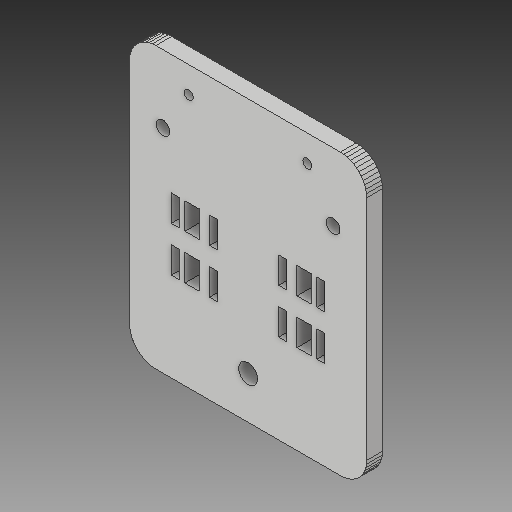
# Autodesk Inventor part: X-Axis-End-Plate
Saved by Autodesk Inventor 2018 (Build 220112000, 112)
## iProperties
Created: 2016-07-20
Part Number: X-Axis-End-Plate
Material: Generic
Document SubType Name: Modeling
Designer: User
Density: 1 g/cm^3
Appearance: Default
Mass: 53.5159 g
Surface Area: 225.376 cm^2
Volume: 53.5159 cm^3
Author: User
Autodesk Inventor part; units mm, degrees
ref_plane "YZ Plane" through (0, 0, 0) normal (1, 0, 0) x (0, 1, 0)
ref_plane "XZ Plane" through (0, 0, 0) normal (0, 1, 0) x (-1, 0, 0)
ref_plane "XY Plane" through (0, 0, 0) normal (0, 0, 1) x (1, 0, 0)
sketch "Sketch1" plane through (0, 0, 0) normal (0, 0, 1) x (1, 0, 0)
  line L0 (481.879114, 151.794374) -> (481.879114, 141.794403)
  line L1 (481.879114, 141.794403) -> (484.879103, 141.794403)
  line L2 (484.879103, 141.794403) -> (484.879103, 151.794374)
  line L3 (484.879103, 151.794374) -> (481.879114, 151.794374)
  line L4 (481.879114, 134.794399) -> (481.879114, 124.794385)
  line L5 (481.879114, 124.794385) -> (484.879103, 124.794385)
  line L6 (484.879103, 124.794385) -> (484.879103, 134.794399)
  line L7 (484.879103, 134.794399) -> (481.879114, 134.794399)
  line L8 (467.379094, 134.794399) -> (467.379094, 124.794385)
  line L9 (467.379094, 124.794385) -> (470.379127, 124.794385)
  line L10 (470.379127, 124.794385) -> (470.379127, 134.794399)
  line L11 (470.379127, 134.794399) -> (467.379094, 134.794399)
  line L12 (472.529125, 134.794399) -> (472.529125, 124.794385)
  line L13 (472.529125, 124.794385) -> (477.929139, 124.794385)
  line L14 (477.929139, 124.794385) -> (477.929139, 134.794399)
  line L15 (477.929139, 134.794399) -> (472.529125, 134.794399)
  line L16 (472.529125, 151.794374) -> (472.529125, 141.794403)
  line L17 (472.529125, 141.794403) -> (477.929139, 141.794403)
  line L18 (477.929139, 141.794403) -> (477.929139, 151.794374)
  line L19 (477.929139, 151.794374) -> (472.529125, 151.794374)
  line L20 (467.379094, 151.794374) -> (467.379094, 141.794403)
  line L21 (467.379094, 141.794403) -> (470.379127, 141.794403)
  line L22 (470.379127, 141.794403) -> (470.379127, 151.794374)
  line L23 (470.379127, 151.794374) -> (467.379094, 151.794374)
  line L24 (541.393546, 188.55966) -> (541.13835, 189.842592)
  line L25 (541.13835, 189.842592) -> (540.717954, 191.081259)
  line L26 (540.717954, 191.081259) -> (540.139367, 192.254387)
  line L27 (540.139367, 192.254387) -> (539.412654, 193.342024)
  line L28 (539.412654, 193.342024) -> (538.550163, 194.325482)
  line L29 (538.550163, 194.325482) -> (537.566754, 195.187911)
  line L30 (537.566754, 195.187911) -> (536.479128, 195.914617)
  line L31 (536.479128, 195.914617) -> (535.30593, 196.493238)
  line L32 (535.30593, 196.493238) -> (534.067263, 196.913635)
  line L33 (534.067263, 196.913635) -> (532.784356, 197.168825)
  line L34 (532.784356, 197.168825) -> (531.479096, 197.254393)
  line L35 (531.479096, 197.254393) -> (461.479063, 197.254393)
  line L36 (461.479063, 197.254393) -> (460.173846, 197.168827)
  line L37 (460.173846, 197.168827) -> (458.890898, 196.913628)
  line L38 (458.890898, 196.913628) -> (457.652231, 196.493231)
  line L39 (457.652231, 196.493231) -> (456.479102, 195.914644)
  line L40 (456.479102, 195.914644) -> (455.391476, 195.187938)
  line L41 (455.391476, 195.187938) -> (454.408051, 194.325477)
  line L42 (454.408051, 194.325477) -> (453.545572, 193.34201)
  line L43 (453.545572, 193.34201) -> (452.818872, 192.254393)
  line L44 (452.818872, 192.254393) -> (452.240268, 191.081231)
  line L45 (452.240268, 191.081231) -> (451.81988, 189.84259)
  line L46 (451.81988, 189.84259) -> (451.564685, 188.559658)
  line L47 (451.564685, 188.559658) -> (451.479117, 187.254397)
  line L48 (451.479117, 187.254397) -> (451.479117, 100.994374)
  line L49 (451.479117, 100.994374) -> (451.564685, 99.689135)
  line L50 (451.564685, 99.689135) -> (451.81988, 98.406203)
  line L51 (451.81988, 98.406203) -> (452.240268, 97.167562)
  line L52 (452.240268, 97.167562) -> (452.818872, 95.994399)
  line L53 (452.818872, 95.994399) -> (453.545572, 94.906782)
  line L54 (453.545572, 94.906782) -> (454.408051, 93.923337)
  line L55 (454.408051, 93.923337) -> (455.391496, 93.060877)
  line L56 (455.391496, 93.060877) -> (456.479122, 92.334171)
  line L57 (456.479122, 92.334171) -> (457.652251, 91.755584)
  line L58 (457.652251, 91.755584) -> (458.890911, 91.335189)
  line L59 (458.890911, 91.335189) -> (460.173864, 91.07999)
  line L60 (460.173864, 91.07999) -> (461.47908, 90.994425)
  line L61 (461.47908, 90.994425) -> (531.479114, 90.994425)
  line L62 (531.479114, 90.994425) -> (532.784373, 91.079994)
  line L63 (532.784373, 91.079994) -> (534.067285, 91.335185)
  line L64 (534.067285, 91.335185) -> (535.306039, 91.755612)
  line L65 (535.306039, 91.755612) -> (536.479237, 92.334233)
  line L66 (536.479237, 92.334233) -> (537.566863, 93.060939)
  line L67 (537.566863, 93.060939) -> (538.550274, 93.923388)
  line L68 (538.550274, 93.923388) -> (539.412743, 94.906843)
  line L69 (539.412743, 94.906843) -> (540.139456, 95.99448)
  line L70 (540.139456, 95.99448) -> (540.71798, 97.167481)
  line L71 (540.71798, 97.167481) -> (541.13843, 98.406304)
  line L72 (541.13843, 98.406304) -> (541.393625, 99.689236)
  line L73 (541.393625, 99.689236) -> (541.47915, 100.993841)
  line L74 (541.47915, 100.993841) -> (541.47915, 187.253864)
  line L75 (541.47915, 187.253864) -> (541.393546, 188.55966)
  line L76 (466.594249, 172.241537) -> (466.344494, 172.844478)
  line L77 (466.344494, 172.844478) -> (465.947221, 173.362246)
  line L78 (465.947221, 173.362246) -> (465.429438, 173.759515)
  line L79 (465.429438, 173.759515) -> (464.826482, 174.009293)
  line L80 (464.826482, 174.009293) -> (464.17945, 174.094495)
  line L81 (464.17945, 174.094495) -> (463.532378, 174.00927)
  line L82 (463.532378, 174.00927) -> (462.929452, 173.759522)
  line L83 (462.929452, 173.759522) -> (462.411649, 173.362223)
  line L84 (462.411649, 173.362223) -> (462.014386, 172.844447)
  line L85 (462.014386, 172.844447) -> (461.764617, 172.241512)
  line L86 (461.764617, 172.241512) -> (461.679408, 171.594428)
  line L87 (461.679408, 171.594428) -> (461.764626, 170.947406)
  line L88 (461.764626, 170.947406) -> (462.014395, 170.344429)
  line L89 (462.014395, 170.344429) -> (462.411658, 169.826674)
  line L90 (462.411658, 169.826674) -> (462.929469, 169.429385)
  line L91 (462.929469, 169.429385) -> (463.532388, 169.179622)
  line L92 (463.532388, 169.179622) -> (464.179462, 169.094414)
  line L93 (464.179462, 169.094414) -> (464.826492, 169.179633)
  line L94 (464.826492, 169.179633) -> (465.429455, 169.429396)
  line L95 (465.429455, 169.429396) -> (465.94723, 169.826675)
  line L96 (465.94723, 169.826675) -> (466.344482, 170.344437)
  line L97 (466.344482, 170.344437) -> (466.594267, 170.947409)
  line L98 (466.594267, 170.947409) -> (466.679473, 171.594468)
  line L99 (466.679473, 171.594468) -> (466.594249, 172.241537)
  line L100 (475.620434, 187.694279) -> (475.450597, 188.104291)
  line L101 (475.450597, 188.104291) -> (475.180424, 188.456408)
  line L102 (475.180424, 188.456408) -> (474.828325, 188.726555)
  line L103 (474.828325, 188.726555) -> (474.418362, 188.896385)
  line L104 (474.418362, 188.896385) -> (473.97834, 188.954328)
  line L105 (473.97834, 188.954328) -> (473.538405, 188.896385)
  line L106 (473.538405, 188.896385) -> (473.128364, 188.726535)
  line L107 (473.128364, 188.726535) -> (472.77627, 188.456381)
  line L108 (472.77627, 188.456381) -> (472.506125, 188.104284)
  line L109 (472.506125, 188.104284) -> (472.336277, 187.694277)
  line L110 (472.336277, 187.694277) -> (472.27834, 187.254297)
  line L111 (472.27834, 187.254297) -> (472.336289, 186.814319)
  line L112 (472.336289, 186.814319) -> (472.506134, 186.404289)
  line L113 (472.506134, 186.404289) -> (472.77627, 186.05222)
  line L114 (472.77627, 186.05222) -> (473.128369, 185.782073)
  line L115 (473.128369, 185.782073) -> (473.538405, 185.612213)
  line L116 (473.538405, 185.612213) -> (473.978345, 185.554281)
  line L117 (473.978345, 185.554281) -> (474.418368, 185.612235)
  line L118 (474.418368, 185.612235) -> (474.828336, 185.782055)
  line L119 (474.828336, 185.782055) -> (475.180429, 186.052209)
  line L120 (475.180429, 186.052209) -> (475.450574, 186.404304)
  line L121 (475.450574, 186.404304) -> (475.620429, 186.81433)
  line L122 (475.620429, 186.81433) -> (475.678374, 187.254369)
  line L123 (475.678374, 187.254369) -> (475.620434, 187.694279)
  line L124 (499.931821, 107.918802) -> (499.575329, 108.779425)
  line L125 (499.575329, 108.779425) -> (499.008238, 109.518518)
  line L126 (499.008238, 109.518518) -> (498.269158, 110.085575)
  line L127 (498.269158, 110.085575) -> (497.408529, 110.442096)
  line L128 (497.408529, 110.442096) -> (496.484906, 110.56372)
  line L129 (496.484906, 110.56372) -> (495.561371, 110.442083)
  line L130 (495.561371, 110.442083) -> (494.700696, 110.085568)
  line L131 (494.700696, 110.085568) -> (493.9616, 109.518475)
  line L132 (493.9616, 109.518475) -> (493.394525, 108.779372)
  line L133 (493.394525, 108.779372) -> (493.03801, 107.918758)
  line L134 (493.03801, 107.918758) -> (492.916389, 106.995156)
  line L135 (492.916389, 106.995156) -> (493.038034, 106.071557)
  line L136 (493.038034, 106.071557) -> (493.394527, 105.210934)
  line L137 (493.394527, 105.210934) -> (493.961618, 104.471842)
  line L138 (493.961618, 104.471842) -> (494.700725, 103.904764)
  line L139 (494.700725, 103.904764) -> (495.561391, 103.548228)
  line L140 (495.561391, 103.548228) -> (496.484929, 103.426615)
  line L141 (496.484929, 103.426615) -> (497.408549, 103.548263)
  line L142 (497.408549, 103.548263) -> (498.269187, 103.904762)
  line L143 (498.269187, 103.904762) -> (499.008255, 104.471834)
  line L144 (499.008255, 104.471834) -> (499.575331, 105.210938)
  line L145 (499.575331, 105.210938) -> (499.931846, 106.071552)
  line L146 (499.931846, 106.071552) -> (500.05347, 106.995179)
  line L147 (500.05347, 106.995179) -> (499.931821, 107.918802)
  line L148 (508.079065, 151.794374) -> (508.079065, 141.794403)
  line L149 (508.079065, 141.794403) -> (511.07914, 141.794403)
  line L150 (511.07914, 141.794403) -> (511.07914, 151.794374)
  line L151 (511.07914, 151.794374) -> (508.079065, 151.794374)
  line L152 (520.621398, 187.694369) -> (520.45156, 188.104381)
  line L153 (520.45156, 188.104381) -> (520.181388, 188.456498)
  line L154 (520.181388, 188.456498) -> (519.829289, 188.726645)
  line L155 (519.829289, 188.726645) -> (519.419326, 188.896475)
  line L156 (519.419326, 188.896475) -> (518.979304, 188.954417)
  line L157 (518.979304, 188.954417) -> (518.539284, 188.896463)
  line L158 (518.539284, 188.896463) -> (518.129316, 188.726644)
  line L159 (518.129316, 188.726644) -> (517.777223, 188.45649)
  line L160 (517.777223, 188.45649) -> (517.507083, 188.1044)
  line L161 (517.507083, 188.1044) -> (517.337241, 187.694408)
  line L162 (517.337241, 187.694408) -> (517.279303, 187.254423)
  line L163 (517.279303, 187.254423) -> (517.337253, 186.814439)
  line L164 (517.337253, 186.814439) -> (517.507092, 186.404425)
  line L165 (517.507092, 186.404425) -> (517.777228, 186.052355)
  line L166 (517.777228, 186.052355) -> (518.129326, 185.782208)
  line L167 (518.129326, 185.782208) -> (518.539289, 185.612378)
  line L168 (518.539289, 185.612378) -> (518.979314, 185.554435)
  line L169 (518.979314, 185.554435) -> (519.419337, 185.61239)
  line L170 (519.419337, 185.61239) -> (519.829305, 185.782209)
  line L171 (519.829305, 185.782209) -> (520.181398, 186.052363)
  line L172 (520.181398, 186.052363) -> (520.451543, 186.404459)
  line L173 (520.451543, 186.404459) -> (520.621398, 186.814485)
  line L174 (520.621398, 186.814485) -> (520.679336, 187.25447)
  line L175 (520.679336, 187.25447) -> (520.621398, 187.694369)
  line L176 (522.579127, 134.794399) -> (522.579127, 124.794385)
  line L177 (522.579127, 124.794385) -> (525.579116, 124.794385)
  line L178 (525.579116, 124.794385) -> (525.579116, 134.794399)
  line L179 (525.579116, 134.794399) -> (522.579127, 134.794399)
  line L180 (522.579127, 151.794374) -> (522.579127, 141.794403)
  line L181 (522.579127, 141.794403) -> (525.579116, 141.794403)
  line L182 (525.579116, 141.794403) -> (525.579116, 151.794374)
  line L183 (525.579116, 151.794374) -> (522.579127, 151.794374)
  line L184 (515.029114, 134.794399) -> (515.029114, 124.794385)
  line L185 (515.029114, 124.794385) -> (520.429129, 124.794385)
  line L186 (520.429129, 124.794385) -> (520.429129, 134.794399)
  line L187 (520.429129, 134.794399) -> (515.029114, 134.794399)
  line L188 (531.194569, 172.24152) -> (530.944815, 172.844461)
  line L189 (530.944815, 172.844461) -> (530.547526, 173.36225)
  line L190 (530.547526, 173.36225) -> (530.029743, 173.759518)
  line L191 (530.029743, 173.759518) -> (529.426786, 174.009297)
  line L192 (529.426786, 174.009297) -> (528.779755, 174.094499)
  line L193 (528.779755, 174.094499) -> (528.132682, 174.009274)
  line L194 (528.132682, 174.009274) -> (527.529793, 173.759541)
  line L195 (527.529793, 173.759541) -> (527.011991, 173.362242)
  line L196 (527.011991, 173.362242) -> (526.614712, 172.844445)
  line L197 (526.614712, 172.844445) -> (526.364949, 172.241525)
  line L198 (526.364949, 172.241525) -> (526.279744, 171.594475)
  line L199 (526.279744, 171.594475) -> (526.364963, 170.947448)
  line L200 (526.364963, 170.947448) -> (526.614726, 170.344486)
  line L201 (526.614726, 170.344486) -> (527.012005, 169.82671)
  line L202 (527.012005, 169.82671) -> (527.529815, 169.429421)
  line L203 (527.529815, 169.429421) -> (528.132698, 169.179673)
  line L204 (528.132698, 169.179673) -> (528.779773, 169.094466)
  line L205 (528.779773, 169.094466) -> (529.426802, 169.179685)
  line L206 (529.426802, 169.179685) -> (530.029765, 169.429448)
  line L207 (530.029765, 169.429448) -> (530.54754, 169.826726)
  line L208 (530.54754, 169.826726) -> (530.944744, 170.344426)
  line L209 (530.944744, 170.344426) -> (531.194529, 170.947397)
  line L210 (531.194529, 170.947397) -> (531.279764, 171.594678)
  line L211 (531.279764, 171.594678) -> (531.194569, 172.24152)
  line L212 (508.079065, 134.794399) -> (508.079065, 124.794385)
  line L213 (508.079065, 124.794385) -> (511.07914, 124.794385)
  line L214 (511.07914, 124.794385) -> (511.07914, 134.794399)
  line L215 (511.07914, 134.794399) -> (508.079065, 134.794399)
  line L216 (515.029114, 151.794374) -> (515.029114, 141.794403)
  line L217 (515.029114, 141.794403) -> (520.429129, 141.794403)
  line L218 (520.429129, 141.794403) -> (520.429129, 151.794374)
  line L219 (520.429129, 151.794374) -> (515.029114, 151.794374)
  point P0 (0, 0)
  constraints: 440 end point, 108 parallel, 86 perpendicular, 7 collinear
extrude "Extrusion1" add sketch "Sketch1" along normal blind 6
sketch "Sketch2" plane through (0, 0, 0) normal (0, 0, -1) x (-1, 0, 0)
  line L0 (-496.484906, 110.56372) -> (-497.408529, 110.442096)
  line L1 (-496.484929, 103.426615) -> (-497.408549, 103.548263)
  line L2 (-496.484906, 110.56372) -> (-496.484929, 103.426615)
  line L3 (-464.17945, 174.094495) -> (-464.826482, 174.009293)
  line L4 (-464.826492, 169.179633) -> (-464.179462, 169.094414)
  line L5 (-464.17945, 174.094495) -> (-464.179462, 169.094414)
  line L6 (-473.538405, 188.896385) -> (-473.97834, 188.954328)
  line L7 (-473.978345, 185.554281) -> (-473.538405, 185.612213)
  line L8 (-473.97834, 188.954328) -> (-473.978345, 185.554281)
  line L9 (-518.979304, 188.954417) -> (-519.419326, 188.896475)
  line L10 (-518.979304, 188.954417) -> (-518.979304, 185.554913)
  line L11 (-529.426786, 174.009297) -> (-528.779755, 174.094499)
  line L12 (-528.779755, 174.094499) -> (-528.779755, 169.095684)
  line L13 (-496.484906, 110.56372) -> (-497.408529, 110.442096)
  line L14 (-496.484929, 103.426615) -> (-497.408549, 103.548263)
  line L15 (-496.484906, 110.56372) -> (-496.484929, 103.426615)
  line L16 (-464.17945, 174.094495) -> (-464.826482, 174.009293)
  line L17 (-464.826492, 169.179633) -> (-464.179462, 169.094414)
  line L18 (-464.17945, 174.094495) -> (-464.179462, 169.094414)
  line L19 (-473.538405, 188.896385) -> (-473.97834, 188.954328)
  line L20 (-473.97834, 185.554281) -> (-473.5384, 185.612213)
  line L21 (-473.97834, 188.954328) -> (-473.97834, 185.554281)
  line L22 (-518.979304, 188.954417) -> (-519.419326, 188.896475)
  line L23 (-518.979304, 188.954417) -> (-518.979304, 185.554913)
  line L24 (-529.426786, 174.009297) -> (-528.779755, 174.094499)
  line L25 (-528.779755, 174.094499) -> (-528.779755, 169.095684)
  point P0 (0, 0)
  point P1 (-518.979304, 187.254665)
  point P2 (-473.97834, 187.254304)
  point P3 (-464.179456, 171.594454)
  point P4 (-528.779755, 171.595092)
  point P5 (-496.484918, 106.995167)
  point P6 (0, 0)
  point P7 (-518.979304, 187.254665)
  point P8 (-473.97834, 187.254304)
  point P9 (-464.179456, 171.594454)
  point P10 (-528.779755, 171.595092)
  point P11 (-496.484918, 106.995167)
  constraints: 36 end point, 10 midpoint, 6 vertical
hole "Hole1" at (518.979304, 187.254665, 0) at (473.97834, 187.254304, 0) at (464.179456, 171.594454, 0) at (528.779755, 171.595092, 0) at (496.484918, 106.995167, 0) direction (0, 0, 1) diameter 3.4 end through all
sketch "Sketch3" plane through (0, 0, 0) normal (0, 0, -1) x (-1, 0, 0)
  line L0 (-496.484906, 110.56372) -> (-497.408529, 110.442096)
  line L1 (-496.484929, 103.426615) -> (-497.408549, 103.548263)
  line L2 (-496.484906, 110.56372) -> (-496.484929, 103.426615)
  line L3 (-464.17945, 174.094495) -> (-464.826482, 174.009293)
  line L4 (-464.826492, 169.179633) -> (-464.179462, 169.094414)
  line L5 (-464.17945, 174.094495) -> (-464.179462, 169.094414)
  line L6 (-473.538405, 188.896385) -> (-473.97834, 188.954328)
  line L7 (-473.97834, 185.554281) -> (-473.5384, 185.612213)
  line L8 (-473.97834, 188.954328) -> (-473.97834, 185.554281)
  line L9 (-518.979304, 188.954417) -> (-519.419326, 188.896475)
  line L10 (-518.979304, 188.954417) -> (-518.979304, 185.554913)
  line L11 (-529.426786, 174.009297) -> (-528.779755, 174.094499)
  line L12 (-528.779755, 174.094499) -> (-528.779755, 169.095684)
  point P0 (0, 0)
  point P1 (0, 0)
  point P2 (-518.979304, 187.254665)
  point P3 (-473.97834, 187.254304)
  point P4 (-464.179456, 171.594454)
  point P5 (-528.779755, 171.595092)
  point P6 (-496.484918, 106.995167)
  constraints: 26 end point, 5 midpoint, 3 vertical
hole "Hole2" at (528.779755, 171.595092, 0) at (464.179456, 171.594454, 0) direction (0, 0, 1) diameter 5.2 end through all
sketch "Sketch4" plane through (0, 0, 0) normal (0, 0, -1) x (-1, 0, 0)
  line L0 (-496.484906, 110.56372) -> (-497.408529, 110.442096)
  line L1 (-496.484929, 103.426615) -> (-497.408549, 103.548263)
  line L2 (-496.484906, 110.56372) -> (-496.484929, 103.426615)
  line L3 (-496.484906, 110.56372) -> (-497.408529, 110.442096)
  line L4 (-496.484929, 103.426615) -> (-497.408549, 103.548263)
  line L5 (-496.484906, 110.56372) -> (-496.484929, 103.426615)
  point P0 (0, 0)
  point P1 (0, 0)
  point P2 (-496.484918, 106.995167)
  point P3 (0, 0)
  point P4 (-496.484918, 106.995167)
  constraints: 12 end point, 2 midpoint
hole "Hole3" at (496.484918, 106.995167, 0) direction (0, 0, 1) diameter 7.2 end through all
body "Solid1"
